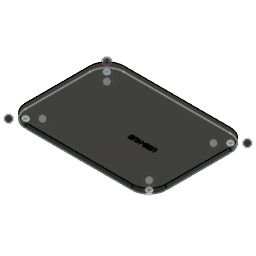
top panel (Autodesk Fusion 360 design; units mm, degrees)
part number: 2026-06-26-18-02-21-889
Autodesk Fusion 360 part; units mm, degrees
note: some values were not read from the file. Set by a fixed rule: the direction of a hole.
sketch "Sketch1" plane through (0, 0, 0) normal (0, 1, 0) x (1, 0, 0)
  line L0 (10, 0) -> (73, 0)
  line L1 (83, -10) -> (83, -48)
  line L2 (73, -58) -> (10, -58)
  line L3 (0, -48) -> (0, -10)
  arc A0 (10, 0) -> (0, -10) centre (10, -10) ccw
  arc A1 (83, -10) -> (73, 0) centre (73, -10) ccw
  arc A2 (0, -48) -> (10, -58) centre (10, -48) ccw
  arc A3 (73, -58) -> (83, -48) centre (73, -48) ccw
  circle A4 centre (5, -5) radius 1.45
  circle A5 centre (78, -5) radius 1.45
  circle A6 centre (78, -53) radius 1.45
  circle A7 centre (5, -53) radius 1.45
  point P0 (83, 0)
  point P1 (0, -58)
  dimension "d1" = 83
  dimension "d2" = 58
  dimension "d3" = 10
  dimension "d4" = 10
  dimension "d5" = 10
  dimension "d8" = 2.9
  dimension "d9" = 2.9
  dimension "d10" = 5
  dimension "d11" = 5
  dimension "d12" = 2.9
  dimension "d13" = 5
  dimension "d14" = 5
  dimension "d15" = 2.9
  dimension "d16" = 5
  dimension "d17" = 5
  constraint horizontal L0
  constraint vertical L1
  constraint horizontal L2
  constraint vertical L3
  constraint coincident origin L0
  constraint coincident origin L3
  constraint tangent L0 A0
  constraint tangent L3 A0
  constraint coincident P0 L0
  constraint coincident P0 L1
  constraint tangent L0 A1
  constraint tangent L1 A1
  constraint coincident P1 L2
  constraint coincident P1 L3
  constraint tangent L2 A2
  constraint tangent L3 A2
  constraint tangent L1 A3
  constraint tangent L2 A3
  constraint equal A2 A3
  measures "d1" distance of origin P0
  measures "d2" distance of origin P1
  measures "d3" radius of A0
  measures "d4" radius of A1
  measures "d5" radius of A2
  measures "d8" diameter of A4
  measures "d9" diameter of A5
  measures "d10" distance of L0 A5.centre
  measures "d11" distance of L1 A5.centre
  measures "d12" diameter of A6
  measures "d13" distance of L1 A6.centre
  measures "d14" distance of L2 A6.centre
  measures "d15" diameter of A7
  measures "d16" distance of L3 A7.centre
  measures "d17" distance of L2 A7.centre
extrude "Extrude1" add sketch "Sketch1" along normal blind 2 contours L0 L1 L2 L3 A0 A1 A2 A3 | A4 | A5 | A6 | A7
extrude "Extrude2" add 1 faces at (31, 2, 38.6667) along direction (0, 1, 0) blind 1
hole "Hole1" at (5, 0, 5) direction (0, 1, 0) diameter 2.9 depth 2 tip angle 118
hole "Hole2" at (5, 0, 53) direction (0, 1, 0) diameter 2.9 depth 2 tip angle 118
hole "Hole3" at (78, 0, 53) direction (0, 1, 0) diameter 2.9 depth 2 tip angle 118
hole "Hole4" at (78, 0, 5) direction (0, 1, 0) diameter 2.9 depth 2 tip angle 118
sketch "Sketch2" plane through (0, 3, 0) normal (0, 1, 0) x (-1, 0, 0)
  arc A0 (0, 48) -> (-10, 58) centre (-10, 48) ccw
  line L0 (-10, 58) -> (-73, 58)
  arc A1 (-73, 58) -> (-83, 48) centre (-73, 48) ccw
  line L1 (-83, 48) -> (-83, 10)
  arc A2 (-83, 10) -> (-73, 0) centre (-73, 10) ccw
  line L2 (-73, 0) -> (-10, 0)
  arc A3 (-10, 0) -> (0, 10) centre (-10, 10) ccw
  line L3 (0, 10) -> (0, 48)
  line L4 (-62.7598, 18.7902) -> (-16.2578, 18.7902) construction
  line L5 (-16.2578, 18.7902) -> (-16.2578, 35.3418) construction
  line L6 (-16.2578, 35.3418) -> (-62.7598, 35.3418) construction
  line L7 (-62.7598, 35.3418) -> (-62.7598, 18.7902) construction
  dimension "d32" = 2.5
  text T0 "USB-HUB" font "Arial" height 2.5 align left top in box 46.5021 x 16.5516 at (-62.7598, 18.7902) x (1, 0) y (0, 1) spacing 1
extrude "Extrude3" cut sketch "Sketch2" against normal blind 0.2 text T0
equation "d33 = 'USB-HUB'"
